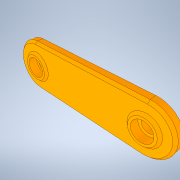
# Autodesk Inventor part: Распорка роликов натяжителя
Saved by Autodesk Inventor 2021.1 (Build 251245010, 245A)
## iProperties
Created: 2026-05-06
Part Number: Распорка роликов натяжителя
Material: Типовые
Document SubType Name: Modeling
Designer: Андрей Тарасов
Density: 1 g/cm^3
Appearance: По умолчанию
Author: Андрей Тарасов
Autodesk Inventor part; units mm, degrees
ref_plane "YZ Plane" through (0, 0, 0) normal (1, 0, 0) x (0, 1, 0)
ref_plane "XZ Plane" through (0, 0, 0) normal (0, 1, 0) x (-1, 0, 0)
ref_plane "XY Plane" through (0, 0, 0) normal (0, 0, 1) x (1, 0, 0)
sketch "Эскиз1" plane through (0, 0, 0) normal (0, 0, 1) x (1, 0, 0)
  line L0 (0, 0) -> (48, 0) construction
  line L1 (0, -10) -> (48, -10)
  line L2 (48, 10) -> (0, 10)
  arc A0 (0, 10) -> (0, -10) centre (0, 0) ccw
  arc A1 (48, -10) -> (48, 10) centre (48, 0) ccw
  circle A2 centre (0, 0) radius 2.8
  circle A3 centre (48, 0) radius 2.8
  point P0 (24, 0)
  dimension "d0" = 48
  dimension "d1" = 20
  dimension "d2" = 5.6
  dimension "d3" = 5.6
  constraints: 8 end point, 4 centre point, 4 point on circle, 4 tangent, 2 coincident, 1 horizontal, 1 midpoint, 1 parallel
  measures "d0" distance of L0.start L0.end
  measures "d1" diameter of A1
  measures "d2" diameter of A2
  measures "d3" diameter of A3
extrude "Выдавливание1" add sketch "Эскиз1" along normal blind 7
chamfer "Фаска1" distance 2 angle 45 2 edges at (-2.8, 0, 0) (45.2, 0, 0)
chamfer "Фаска2" distance 3.5 angle 45 4 edges at (24, 10, 0) (-10, 0, 0) (24, -10, 0) (58, 0, 0)
sketch "Эскиз3" plane through (0, 0, 7) normal (0, 0, 1) x (1, 0, 0)
  circle A0 centre (0, 0) radius 5
  circle A1 centre (48, 0) radius 5
  circle A2 centre (0, 0) radius 2.8 projected
  circle A3 centre (48, 0) radius 2.8 projected
  dimension "d19" = 10
  constraints: 2 centre point, 2 coincident, 1 equal radius
  measures "d19" diameter of A0
extrude "Выдавливание3" add sketch "Эскиз3" along normal blind 1
chamfer "Фаска4" distance 1 angle 45 6 edges at (24, 10, 7) (-10, 0, 7) (24, -10, 7) (58, 0, 7) (43, 0, 7) (-5, 0, 7)
sketch "Эскиз4" plane through (0, 0, 8) normal (0, 0, 1) x (1, 0, 0)
  circle A0 centre (0, 0) radius 4
  circle A1 centre (48, 0) radius 2.8 projected
  circle A2 centre (48, 0) radius 4
  dimension "d26" = 8
  constraints: 2 centre point, 2 coincident, 1 equal radius
  measures "d26" diameter of A0
extrude "Выдавливание4" cut sketch "Эскиз4" against normal blind 3.5 contours A0 | A1 | A2
